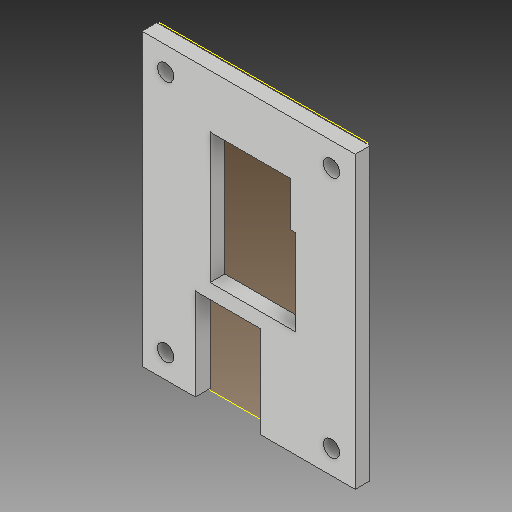
# Autodesk Inventor part: Pieza4
Saved by Autodesk Inventor 2017 (Build 210142000, 142)
## iProperties
Part Number: Pieza4
Material: Genérico
Document SubType Name: Modeling
Designer: user
Density: 1 g/cm^3
Appearance: Valor por defecto
Author: user
Autodesk Inventor part; units mm, degrees
ref_plane "YZ Plane" through (0, 0, 0) normal (1, 0, 0) x (0, 1, 0)
ref_plane "XZ Plane" through (0, 0, 0) normal (0, 1, 0) x (-1, 0, 0)
ref_plane "XY Plane" through (0, 0, 0) normal (0, 0, 1) x (1, 0, 0)
ref_plane "Plano de trabajo1" through (0, 0, 0) normal (0, 0, 1) x (1, 0, 0)
sketch "Boceto1" plane through (0, 0, 0) normal (0, 0, 1) x (1, 0, 0)
  line L0 (-15, -30) -> (3, -30) projected
  line L1 (3, -30) -> (3, -19) projected
  line L2 (3, -19) -> (-15, -19) projected
  line L3 (-15, -19) -> (-15, -30) projected
  line L4 (-12, -12) -> (-7, -12) projected
  line L5 (-7, 15) -> (-12, 15) projected
  line L6 (-12, 15) -> (-12, -12) projected
  line L7 (-12, 30) -> (-12, 16) projected
  line L8 (-12, 16) -> (13, 16) projected
  line L9 (13, 16) -> (13, 30) projected
  line L10 (13, 30) -> (-12, 30) projected
  line L11 (-15, -30) -> (-15, -19) projected
  line L12 (-15, -19) -> (3, -19) projected
  line L13 (3, -19) -> (3, -30) projected
  line L14 (3, -30) -> (-15, -30) projected
  line L15 (-12, -12) -> (-12, 15) projected
  line L16 (-12, 15) -> (15, 15) projected
  line L17 (15, 15) -> (15, -12) projected
  line L18 (15, -12) -> (-12, -12) projected
  line L19 (-12, 30) -> (13, 30) projected
  line L20 (13, 30) -> (13, 16) projected
  line L21 (13, 16) -> (-12, 16) projected
  line L22 (-12, 16) -> (-12, 30) projected
  line L23 (-22, 35) -> (-22, -35) projected
  line L24 (-22, -35) -> (22, -35) projected
  line L25 (22, -35) -> (22, 35) projected
  line L26 (22, 35) -> (-22, 35) projected
  line L27 (-22, -35) -> (-22, 35) projected
  line L28 (-22, 35) -> (22, 35) projected
  line L29 (22, 35) -> (22, -35) projected
  line L30 (22, -35) -> (-22, -35) projected
  line L31 (-36, -49) -> (36, -49) projected
  line L32 (36, -49) -> (36, 49) projected
  line L33 (36, 49) -> (-36, 49) projected
  line L34 (-36, 49) -> (-36, -49) projected
  line L35 (36, -49) -> (36, 49)
  line L36 (36, 49) -> (-36, 49)
  line L37 (-36, 49) -> (-36, -49)
  line L38 (22, -35) -> (4, -35)
  line L39 (4, -35) -> (4, -18)
  line L40 (15, 15) -> (-12, 15)
  line L41 (-12, 15) -> (-12, -12)
  line L42 (-12, -12) -> (15, -12)
  line L43 (15, -12) -> (15, 15)
  line L44 (-13, -13) -> (-13, 16)
  line L45 (-13, 16) -> (16, 16)
  line L46 (16, 16) -> (16, -13)
  line L47 (16, -13) -> (-13, -13)
  line L48 (13, 16) -> (-8, 16)
  line L49 (-13, 16) -> (14, 16)
  line L50 (14, 16) -> (14, 31)
  line L51 (14, 31) -> (-13, 31)
  line L52 (-13, 31) -> (-13, 16)
  line L53 (4, -18) -> (-18, -18)
  line L54 (-18, -18) -> (-18, -49)
  line L55 (4, -35) -> (4, -49)
  line L56 (-36, -49) -> (-18, -49)
  line L57 (4, -49) -> (36, -49)
  line L58 (-7, -12) -> (-7, 15) projected
  circle A0 centre (28, -41) radius 2.75 projected
  circle A1 centre (-28, 41) radius 2.75 projected
  circle A2 centre (28, 41) radius 2.75 projected
  circle A3 centre (-28, -41) radius 2.75 projected
  point P0 (0, 0)
  dimension "d0" = 18
  dimension "d1" = 17
  dimension "d2" = 1
  dimension "d4" = 27
  dimension "d5" = 15
  dimension "d6" = 22
  dimension "d7" = 90
  dimension "d8" = 98
  dimension "d9" = 44
  constraints: 46 end point, 9 parallel, 8 perpendicular, 5 horizontal, 1 point on line, 3 other
  measures "d0" distance of L24.end L38.end
  measures "d1" distance of L38.end L39.end
  measures "d2" distance between parallel lines of L41 L44
  measures "d4" distance of L50.end L51.end
  measures "d5" distance of L49.end L50.end
  measures "d6" distance of L39.end L53.end
  measures "d7" angle of L25 L48
  measures "d8" distance between parallel lines of L33 L57
  measures "d9" distance from line of L48.end L32
extrude "Extrusión1" add sketch "Boceto1" along normal blind 5 contours L26 L25 L24 L39 L53 L54 L23 | L23 L24 L54 L31 L34 L33 L32 L55 L25 L26 | A0 | A1 | A2 | A3
sketch "Boceto2" plane through (0, 0, 5) normal (0, 0, 1) x (1, 0, 0)
  point P0 (-28, 41)
  point P1 (28, 41)
  point P2 (28, -41)
  point P3 (-28, -41)
hole "Agujero1" at (-28, 41, 5) at (28, 41, 5) at (28, -41, 5) at (-28, -41, 5) direction (0, 0, -1) diameter 5.5 depth 5
